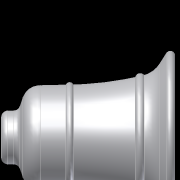
# Autodesk Inventor part: Glocke01
Saved by Autodesk Inventor 2013 (Build 170138000, 138)
## iProperties
Created: 2005-03-09
Part Number: Glocke01
Document SubType Name: Modeling
Designer: acad
Manufacturer: Standard
Standards Organization: Custom
Material: Allgemein
Density: 1 g/cm^3
Author: acad
Autodesk Inventor part; units mm, degrees
ref_plane "YZ Plane" through (0, 0, 0) normal (1, 0, 0) x (0, 1, 0)
ref_plane "XZ Plane" through (0, 0, 0) normal (0, 1, 0) x (-1, 0, 0)
ref_plane "XY Plane" through (0, 0, 0) normal (0, 0, 1) x (1, 0, 0)
sketch "Skizze1" plane through (0, 0, 0) normal (0, 0, 1) x (1, 0, 0)
  line L0 (-3.4404, 0) -> (70.0911, 0)
  line L1 (0, 0) -> (0, 6.4889)
  arc A0 (2, 8.4889) -> (0, 6.4889) centre (2, 6.4889) ccw
  line L2 (2, 8.4889) -> (4, 8.4889)
  arc A1 (4, 8.4889) -> (5.892, 9.8407) centre (4, 10.4889) ccw
  line L3 (5.892, 9.8407) -> (6.8724, 12.7022)
  arc A2 (12.477, 16.4802) -> (6.8724, 12.7022) centre (12.172, 10.8866) ccw
  line L4 (12.477, 16.4802) -> (21.8918, 16.6762)
  arc A3 (21.8918, 16.6762) -> (44.8462, 19.6376) centre (20.1446, 120.6615) ccw
  arc A4 (44.8462, 19.6376) -> (50.0078, 23.3456) centre (42.8273, 27.8944) ccw
  line L5 (50.0078, 23.3456) -> (52.126, 26.6894)
  arc A5 (53.3931, 24.3866) -> (52.126, 26.6894) centre (53.3931, 25.8866) ccw
  line L6 (53.3931, 24.3866) -> (52.8896, 24.3866)
  line L7 (7.2835, 5.2734) -> (8.0875, 10.76)
  arc A6 (12.7191, 14.8474) -> (8.0875, 10.76) centre (12.8186, 10.0668) ccw
  arc A7 (20.5314, 15.01) -> (46.5295, 18.2563) centre (19.9979, 125.0087) ccw
  arc A8 (46.5295, 18.2563) -> (51.2062, 21.7968) centre (43.0974, 27.6489) ccw
  line L8 (51.2062, 21.7968) -> (52.8896, 24.3866)
  line L9 (7.2835, 5.2734) -> (7.2835, 0)
  line L10 (20.5314, 15.01) -> (12.7191, 14.8474)
  arc A9 (45.157, 19.7199) -> (42.2987, 19.0486) centre (43.8734, 18.7648) ccw
  arc A10 (22.8074, 16.6956) -> (20.3993, 16.6451) centre (21.6136, 16.181) ccw
  point P0 (23.9468, 16.731)
  point P1 (26.5001, 16.8559)
  dimension "d1" = 1.5
  dimension "d5" = 8.5
  dimension "d6" = 10
  dimension "d14" = 2
  dimension "d15" = 2
  dimension "d16" = 1.6
  dimension "d23" = 110
  dimension "d24" = 104
  dimension "d26" = 1.3
  constraints: 27 point on circle, 22 end point, 11 centre point, 10 tangent, 3 perpendicular, 3 point on line, 2 parallel, 1 horizontal
  measures "d1" radius of A5
  measures "d5" radius of A4
  measures "d6" radius of A8
  measures "d14" radius of A1
  measures "d15" radius of A0
  measures "d16" radius of A9
  measures "d23" radius of A7
  measures "d24" radius of A3
  measures "d26" radius of A10
revolve "Drehung3" add sketch "Skizze1" angle 360 about axis through (-3.4404, 0, 0) along (1, 0, 0)
sketch "Skizze2" plane through (0, 0, 0) normal (-1, 0, 0) x (0, 0, 1)
  circle A0 centre (0, 0) radius 6.4889 projected
  constraints: 1 coincident
hole "Bohrung1" at (0, 0, 0) direction (1, 0, 0) diameter 4.917 end through all thread size "M6x1" class "6H" standard "ANSI Metrisches M Profil"
